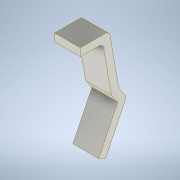
# Autodesk Inventor part: Button_leg
Saved by Autodesk Inventor 2020 (Build 240168000, 168)
## iProperties
Created: 2019-08-05
Part Number: Button_leg
Material: Silver
Document SubType Name: Modeling
Designer: Yusuf
Mass: 0.0166325 g
Surface Area: 0.14232 cm^2
Volume: 0.00158556 cm^3
Density: 10.49 g/cm^3
Appearance: Silver
Author: Yusuf
Autodesk Inventor part; units mm, degrees
ref_plane "YZ Plane" through (0, 0, 0) normal (1, 0, 0) x (0, 1, 0)
ref_plane "XZ Plane" through (0, 0, 0) normal (0, 1, 0) x (-1, 0, 0)
ref_plane "XY Plane" through (0, 0, 0) normal (0, 0, 1) x (1, 0, 0)
sketch "Sketch1" plane through (0, 0, 0) normal (1, 0, 0) x (0, 1, 0)
  line L0 (0, -0.8453) -> (1.6, -1.6232)
  line L1 (1.6, -1.6232) -> (2, -1.3527)
  line L2 (2, -1.3527) -> (4, -1)
  line L3 (4, -1) -> (4, 0)
  point P0 (0, 0)
  dimension "d0" = 4
  dimension "d1" = 1
  dimension "d2" = 2
  dimension "d3" = 0.4
  dimension "d4" = 120
  dimension "d5" = 100
  constraints: 8 end point, 1 horizontal alignment, 1 point on line, 1 vertical, 1 vertical alignment
  measures "d0" horizontal distance of L0.start L3.end
  measures "d1" distance of L2.end L3.end
  measures "d2" horizontal distance of L1.end L2.end
  measures "d3" horizontal distance of L0.end L1.end
  measures "d4" angle of L1 L0
  measures "d5" angle of L3 L2
sketch "Sketch2" plane through (0, 0, 0) normal (0, 0, 1) x (1, 0, 0)
  line L0 (-0.5, 3.85) -> (0.5, 3.85)
  line L1 (0.5, 3.85) -> (0.5, 4.15)
  line L2 (0.5, 4.15) -> (-0.5, 4.15)
  line L3 (-0.5, 4.15) -> (-0.5, 3.85)
  line L4 (-0.5, 3.85) -> (0.5, 4.15) construction
  line L5 (0.5, 3.85) -> (-0.5, 4.15) construction
  point P0 (0, 0)
  point P1 (0, 4)
  dimension "d6" = 1
  dimension "d7" = 0.3
  constraints: 12 end point, 2 midpoint, 2 parallel, 1 horizontal, 1 perpendicular
  measures "d6" distance of L2.end L1.end
  measures "d7" distance of L1.end L0.end
sweep "Sweep1" add profiles "Sketch2" path "Sketch1" path curves L3 L2 L1 L0
chamfer "Chamfer1" distance 0.1 angle 45 4 edges at (0, 4.15, -1.1259) (0, 2.0575, -1.4948) (0, 1.6123, -1.796) (0, 3.85, -0.8741)
body "Solid1"
